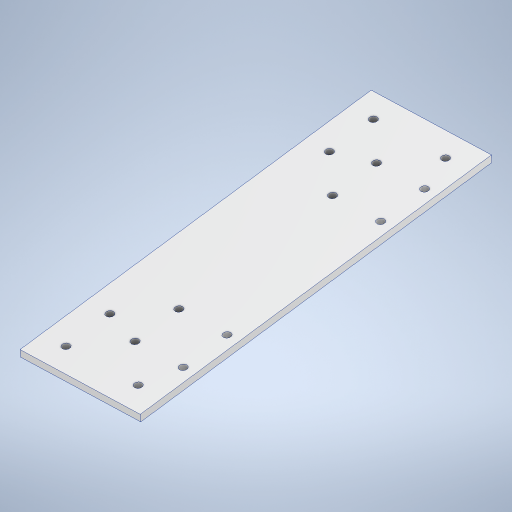
# Autodesk Inventor part: frontPlate
Saved by Autodesk Inventor 2024 (Build 280153000, 153)
## iProperties
Created: 2023-10-26
Part Number: frontPlate
Material: アルミニウム 6061
Document SubType Name: Modeling
Designer: jwith
Density: 2.7 g/cm^3
Appearance: アルミニウム - フラット
Mass: 63.888 g
Surface Area: 174.57 cm^2
Volume: 23.6622 cm^3
Author: jwith
Autodesk Inventor part; units mm, degrees
ref_plane "YZ Plane" through (0, 0, 0) normal (1, 0, 0) x (0, 1, 0)
ref_plane "XZ Plane" through (0, 0, 0) normal (0, 1, 0) x (-1, 0, 0)
ref_plane "XY Plane" through (0, 0, 0) normal (0, 0, 1) x (1, 0, 0)
sketch "スケッチ1" plane through (0, 0, 0) normal (0, 0, 1) x (1, 0, 0)
  line L0 (0, 0) -> (160, 0)
  line L1 (160, 0) -> (160, 50)
  line L2 (160, 50) -> (0, 50)
  line L3 (0, 50) -> (0, 0)
  dimension "d0" = 160
  dimension "d1" = 50
  constraints: 8 end point, 2 parallel, 1 horizontal, 1 perpendicular
  measures "d0" distance of L1.end L2.end
  measures "d1" distance of L0.end L1.end
extrude "押し出し1" add sketch "スケッチ1" against normal blind 3
sketch "スケッチ2" plane through (0, 0, 0) normal (0, 0, 1) x (1, 0, 0)
  line L0 (160, 50) -> (0, 50) projected
  line L1 (160, 0) -> (160, 50) projected
  line L2 (0, 50) -> (0, 0) projected
  line L3 (0, 0) -> (160, 0) projected
  point P0 (135, 45)
  point P1 (135, 25)
  point P2 (25, 45)
  point P3 (25, 25)
  point P4 (115, 45)
  point P5 (115, 25)
  point P6 (45, 45)
  point P7 (45, 25)
  point P8 (150, 40)
  point P9 (150, 10)
  point P10 (10, 40)
  point P11 (10, 10)
  dimension "d4" = 5
  dimension "d5" = 25
  dimension "d6" = 20
  dimension "d7" = 5
  dimension "d8" = 25
  dimension "d9" = 20
  dimension "d10" = 20
  dimension "d11" = 20
  dimension "d12" = 10
  dimension "d13" = 10
  dimension "d14" = 10
  dimension "d15" = 10
  dimension "d16" = 20
  dimension "d17" = 5
  dimension "d18" = 5
  dimension "d19" = 20
  measures "d4" distance from line of L0 point (135, 45)
  measures "d5" distance from line of L1 point (135, 45)
  measures "d6" distance of point (135, 45) point (135, 25)
  measures "d7" distance from line of L0 point (25, 45)
  measures "d8" distance from line of L2 point (25, 45)
  measures "d9" distance of point (25, 45) point (25, 25)
  measures "d10" distance of point (115, 45) point (135, 45)
  measures "d11" distance of point (25, 45) point (45, 45)
  measures "d12" distance from line of L1 point (150, 40)
  measures "d13" distance from line of L3 point (150, 10)
  measures "d14" distance from line of L2 point (10, 40)
  measures "d15" distance from line of L3 point (10, 10)
  measures "d16" distance of point (45, 45) point (45, 25)
  measures "d17" distance from line of L0 point (45, 45)
  measures "d18" distance from line of L0 point (115, 45)
  measures "d19" distance of point (115, 45) point (115, 25)
hole "穴1" at (135, 45, 0) at (135, 25, 0) at (25, 45, 0) at (25, 25, 0) at (115, 45, 0) at (115, 25, 0) at (45, 45, 0) at (45, 25, 0) at (150, 40, 0) at (150, 10, 0) at (10, 40, 0) at (10, 10, 0) direction (0, 0, -1) diameter 3.2 end through all
sketch "スケッチ3" plane through (0, 0, 0) normal (0, 0, 1) x (1, 0, 0)
  line L0 (0, 0) -> (160, 0) projected
  line L1 (0, 50) -> (0, 0) projected
  line L2 (160, 0) -> (160, 50) projected
  point P0 (30, 10)
  point P1 (130, 10)
  dimension "d27" = 10
  dimension "d28" = 30
  dimension "d29" = 10
  dimension "d30" = 30
  measures "d27" distance from line of L0 point (30, 10)
  measures "d28" distance from line of L1 point (30, 10)
  measures "d29" distance from line of L0 point (130, 10)
  measures "d30" distance from line of L2 point (130, 10)
hole "穴2" at (30, 10, 0) at (130, 10, 0) direction (0, 0, -1) diameter 3.2 end through all
